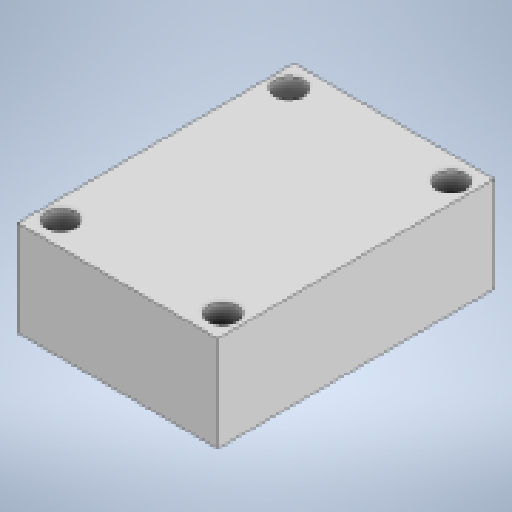
# Autodesk Inventor part: Servo_Driver
Saved by Autodesk Inventor 2025.2 (Build 292293000, 293)
## iProperties
Created: 2025-05-14
Part Number: Servo_Driver
Material: Generic
Document SubType Name: Modeling
Designer: chris
Density: 1 g/cm^3
Appearance: Default
Author: chris
Autodesk Inventor part; units mm, degrees
ref_plane "YZ Plane" through (0, 0, 0) normal (1, 0, 0) x (0, 1, 0)
ref_plane "XZ Plane" through (0, 0, 0) normal (0, 1, 0) x (-1, 0, 0)
ref_plane "XY Plane" through (0, 0, 0) normal (0, 0, 1) x (1, 0, 0)
sketch "Sketch1" plane through (0, 0, 0) normal (0, 1, 0) x (-1, 0, 0)
  line L0 (0, 0) -> (42, 0)
  line L1 (42, 0) -> (42, -58)
  line L2 (42, -58) -> (0, -58)
  line L3 (0, -58) -> (0, 0)
  dimension "d0" = 58
  dimension "d1" = 42
  constraints: 8 end point, 2 parallel, 1 horizontal, 1 perpendicular
  measures "d0" distance of L0.end L1.end
  measures "d1" distance of L1.end L2.end
extrude "Extrusion1" add sketch "Sketch1" along normal blind 20
sketch "Sketch2" plane through (0, 20, 0) normal (0, 1, 0) x (1, 0, 0)
  line L0 (-29.2926, 35.5201) -> (-17.3649, 35.5201) construction
  line L1 (-17.3649, 35.5201) -> (-17.3649, 9.1969) construction
  line L2 (-17.3649, 9.1969) -> (-29.2926, 9.1969) construction
  line L3 (-29.2926, 9.1969) -> (-29.2926, 35.5201) construction
  spline S0 degree 2 poles (-27.9624, 31.884) (-28.3424, 31.884) (-28.8757, 32.0428) (-29.1111, 32.1562) knots 0 0 0 1 2 2 2
  line L4 (-29.1111, 32.1562) -> (-29.1111, 32.7405)
  line L5 (-29.1111, 32.7405) -> (-29.077, 32.7405)
  spline S1 degree 2 poles (-29.077, 32.7405) (-28.8473, 32.525) (-28.2658, 32.2867) (-27.9964, 32.2867) knots 0 0 0 1 2 2 2
  spline S2 degree 2 poles (-27.9964, 32.2867) (-27.6107, 32.2867) (-27.2164, 32.6072) (-27.2164, 32.871) knots 0 0 0 1 2 2 2
  spline S3 degree 2 poles (-27.2164, 32.871) (-27.2164, 33.0809) (-27.4235, 33.3418) (-27.6475, 33.4071) knots 0 0 0 1 2 2 2
  spline S4 degree 2 poles (-27.6475, 33.4071) (-27.8092, 33.4524) (-28.0787, 33.5148) (-28.28, 33.5659) knots 0 0 0 1 2 2 2
  spline S5 degree 2 poles (-28.28, 33.5659) (-28.4616, 33.6141) (-28.748, 33.7588) (-28.8586, 33.875) knots 0 0 0 1 2 2 2
  spline S6 degree 2 poles (-28.8586, 33.875) (-28.9664, 33.9913) (-29.0855, 34.3033) (-29.0855, 34.5075) knots 0 0 0 1 2 2 2
  spline S7 degree 2 poles (-29.0855, 34.5075) (-29.0855, 34.933) (-28.4218, 35.5088) (-27.9085, 35.5088) knots 0 0 0 1 2 2 2
  spline S8 degree 2 poles (-27.9085, 35.5088) (-27.6135, 35.5088) (-27.0916, 35.3925) (-26.8675, 35.2819) knots 0 0 0 1 2 2 2
  line L6 (-26.8675, 35.2819) -> (-26.8675, 34.7259)
  line L7 (-26.8675, 34.7259) -> (-26.9016, 34.7259)
  spline S9 degree 2 poles (-26.9016, 34.7259) (-27.0689, 34.8791) (-27.5908, 35.106) (-27.8773, 35.106) knots 0 0 0 1 2 2 2
  spline S10 degree 2 poles (-27.8773, 35.106) (-28.2006, 35.106) (-28.6005, 34.8025) (-28.6005, 34.5558) knots 0 0 0 1 2 2 2
  spline S11 degree 2 poles (-28.6005, 34.5558) (-28.6005, 34.3345) (-28.3651, 34.0707) (-28.1439, 34.0112) knots 0 0 0 1 2 2 2
  spline S12 degree 2 poles (-28.1439, 34.0112) (-27.9964, 33.9715) (-27.5681, 33.8694) (-27.4263, 33.8268) knots 0 0 0 1 2 2 2
  spline S13 degree 2 poles (-27.4263, 33.8268) (-27.0661, 33.7162) (-26.7314, 33.2709) (-26.7314, 32.9447) knots 0 0 0 1 2 2 2
  spline S14 degree 2 poles (-26.7314, 32.9447) (-26.7314, 32.7377) (-26.8987, 32.3406) (-27.0491, 32.2016) knots 0 0 0 1 2 2 2
  spline S15 degree 2 poles (-27.0491, 32.2016) (-27.2164, 32.0485) (-27.6419, 31.884) (-27.9624, 31.884) knots 0 0 0 1 2 2 2
  line L8 (-26.2577, 31.9464) -> (-26.2577, 35.4464)
  line L9 (-26.2577, 35.4464) -> (-24.0681, 35.4464)
  line L10 (-24.0681, 35.4464) -> (-24.0681, 35.0323)
  line L11 (-24.0681, 35.0323) -> (-25.7926, 35.0323)
  line L12 (-25.7926, 35.0323) -> (-25.7926, 34.0736)
  line L13 (-25.7926, 34.0736) -> (-24.1844, 34.0736)
  line L14 (-24.1844, 34.0736) -> (-24.1844, 33.6595)
  line L15 (-24.1844, 33.6595) -> (-25.7926, 33.6595)
  line L16 (-25.7926, 33.6595) -> (-25.7926, 32.3605)
  line L17 (-25.7926, 32.3605) -> (-24.0681, 32.3605)
  line L18 (-24.0681, 32.3605) -> (-24.0681, 31.9464)
  line L19 (-24.0681, 31.9464) -> (-26.2577, 31.9464)
  line L20 (-20.8489, 31.9464) -> (-21.453, 31.9464)
  line L21 (-21.453, 31.9464) -> (-22.5592, 33.339)
  line L22 (-22.5592, 33.339) -> (-23.0924, 33.339)
  line L23 (-23.0924, 33.339) -> (-23.0924, 31.9464)
  line L24 (-23.0924, 31.9464) -> (-23.5576, 31.9464)
  line L25 (-23.5576, 31.9464) -> (-23.5576, 35.4464)
  line L26 (-23.5576, 35.4464) -> (-22.6556, 35.4464)
  spline S16 degree 2 poles (-22.6556, 35.4464) (-22.355, 35.4464) (-21.9494, 35.3811) (-21.765, 35.262) knots 0 0 0 1 2 2 2
  spline S17 degree 2 poles (-21.765, 35.262) (-21.5807, 35.1429) (-21.368, 34.7713) (-21.368, 34.4962) knots 0 0 0 1 2 2 2
  spline S18 degree 2 poles (-21.368, 34.4962) (-21.368, 34.1133) (-21.7594, 33.5943) (-22.094, 33.4695) knots 0 0 0 1 2 2 2
  line L27 (-22.094, 33.4695) -> (-20.8489, 31.9464)
  spline S19 degree 2 poles (-21.853, 34.4593) (-21.853, 34.6125) (-21.9607, 34.8479) (-22.0742, 34.9245) knots 0 0 0 1 2 2 2
  spline S20 degree 2 poles (-22.0742, 34.9245) (-22.1735, 34.9897) (-22.4372, 35.0436) (-22.6301, 35.0436) knots 0 0 0 1 2 2 2
  line L28 (-22.6301, 35.0436) -> (-23.0924, 35.0436)
  line L29 (-23.0924, 35.0436) -> (-23.0924, 33.7276)
  line L30 (-23.0924, 33.7276) -> (-22.684, 33.7276)
  spline S21 degree 2 poles (-22.684, 33.7276) (-22.4826, 33.7276) (-22.1621, 33.7985) (-22.0515, 33.9091) knots 0 0 0 1 2 2 2
  spline S22 degree 2 poles (-22.0515, 33.9091) (-21.9494, 34.0055) (-21.853, 34.2778) (-21.853, 34.4593) knots 0 0 0 1 2 2 2
  line L31 (-18.0325, 35.4464) -> (-19.2379, 31.9464)
  line L32 (-19.2379, 31.9464) -> (-19.7399, 31.9464)
  line L33 (-19.7399, 31.9464) -> (-20.9453, 35.4464)
  line L34 (-20.9453, 35.4464) -> (-20.4462, 35.4464)
  line L35 (-20.4462, 35.4464) -> (-19.4761, 32.5391)
  line L36 (-19.4761, 32.5391) -> (-18.5061, 35.4464)
  line L37 (-18.5061, 35.4464) -> (-18.0325, 35.4464)
  spline S23 degree 2 poles (-15.2217, 35.0464) (-15.0231, 34.8139) (-14.8019, 34.1331) (-14.8019, 33.6964) knots 0 0 0 1 2 2 2
  spline S24 degree 2 poles (-14.8019, 33.6964) (-14.8019, 33.2709) (-15.0175, 32.5817) (-15.2217, 32.3491) knots 0 0 0 1 2 2 2
  spline S25 degree 2 poles (-15.2217, 32.3491) (-15.4372, 32.1052) (-16.0073, 31.8726) (-16.3505, 31.8726) knots 0 0 0 1 2 2 2
  spline S26 degree 2 poles (-16.3505, 31.8726) (-16.7051, 31.8726) (-17.2723, 32.1137) (-17.4794, 32.3491) knots 0 0 0 1 2 2 2
  spline S27 degree 2 poles (-17.4794, 32.3491) (-17.6808, 32.5817) (-17.8963, 33.2652) (-17.8963, 33.6964) knots 0 0 0 1 2 2 2
  spline S28 degree 2 poles (-17.8963, 33.6964) (-17.8963, 34.136) (-17.6779, 34.8054) (-17.4765, 35.0464) knots 0 0 0 1 2 2 2
  spline S29 degree 2 poles (-17.4765, 35.0464) (-17.2723, 35.279) (-16.7022, 35.5201) (-16.3505, 35.5201) knots 0 0 0 1 2 2 2
  spline S30 degree 2 poles (-16.3505, 35.5201) (-15.9932, 35.5201) (-15.4202, 35.2705) (-15.2217, 35.0464) knots 0 0 0 1 2 2 2
  spline S31 degree 2 poles (-15.2869, 33.6964) (-15.2869, 34.0424) (-15.4372, 34.5784) (-15.5734, 34.7543) knots 0 0 0 1 2 2 2
  spline S32 degree 2 poles (-15.5734, 34.7543) (-15.7124, 34.9358) (-16.1038, 35.1173) (-16.3477, 35.1173) knots 0 0 0 1 2 2 2
  spline S33 degree 2 poles (-16.3477, 35.1173) (-16.6001, 35.1173) (-16.9802, 34.9415) (-17.1248, 34.7543) knots 0 0 0 1 2 2 2
  spline S34 degree 2 poles (-17.1248, 34.7543) (-17.2638, 34.5756) (-17.4113, 34.0367) (-17.4113, 33.6964) knots 0 0 0 1 2 2 2
  spline S35 degree 2 poles (-17.4113, 33.6964) (-17.4113, 33.0071) (-16.8327, 32.2754) (-16.3477, 32.2754) knots 0 0 0 1 2 2 2
  spline S36 degree 2 poles (-16.3477, 32.2754) (-15.8627, 32.2754) (-15.2869, 33.0071) (-15.2869, 33.6964) knots 0 0 0 1 2 2 2
  spline S37 degree 2 poles (-26.1783, 27.9309) (-26.1783, 27.4515) (-26.5669, 26.6801) (-26.8931, 26.4645) knots 0 0 0 1 2 2 2
  spline S38 degree 2 poles (-26.8931, 26.4645) (-27.1597, 26.2972) (-27.7071, 26.1837) (-28.1325, 26.1837) knots 0 0 0 1 2 2 2
  line L38 (-28.1325, 26.1837) -> (-28.9381, 26.1837)
  line L39 (-28.9381, 26.1837) -> (-28.9381, 29.6837)
  line L40 (-28.9381, 29.6837) -> (-28.141, 29.6837)
  spline S39 degree 2 poles (-28.141, 29.6837) (-27.6475, 29.6837) (-27.0859, 29.5362) (-26.8874, 29.4057) knots 0 0 0 1 2 2 2
  spline S40 degree 2 poles (-26.8874, 29.4057) (-26.5499, 29.1817) (-26.1783, 28.4414) (-26.1783, 27.9309) knots 0 0 0 1 2 2 2
  spline S41 degree 2 poles (-26.6633, 27.9365) (-26.6633, 28.3393) (-26.9299, 28.9094) (-27.1937, 29.0711) knots 0 0 0 1 2 2 2
  spline S42 degree 2 poles (-27.1937, 29.0711) (-27.3809, 29.1817) (-27.8035, 29.2809) (-28.1184, 29.2809) knots 0 0 0 1 2 2 2
  line L41 (-28.1184, 29.2809) -> (-28.4729, 29.2809)
  line L42 (-28.4729, 29.2809) -> (-28.4729, 26.5865)
  line L43 (-28.4729, 26.5865) -> (-28.1184, 26.5865)
  spline S43 degree 2 poles (-28.1184, 26.5865) (-27.8092, 26.5865) (-27.3412, 26.6857) (-27.1512, 26.819) knots 0 0 0 1 2 2 2
  spline S44 degree 2 poles (-27.1512, 26.819) (-26.9073, 26.9835) (-26.6633, 27.5281) (-26.6633, 27.9365) knots 0 0 0 1 2 2 2
  line L44 (-22.9648, 26.1837) -> (-23.5689, 26.1837)
  line L45 (-23.5689, 26.1837) -> (-24.6751, 27.5763)
  line L46 (-24.6751, 27.5763) -> (-25.2083, 27.5763)
  line L47 (-25.2083, 27.5763) -> (-25.2083, 26.1837)
  line L48 (-25.2083, 26.1837) -> (-25.6735, 26.1837)
  line L49 (-25.6735, 26.1837) -> (-25.6735, 29.6837)
  line L50 (-25.6735, 29.6837) -> (-24.7715, 29.6837)
  spline S45 degree 2 poles (-24.7715, 29.6837) (-24.4709, 29.6837) (-24.0653, 29.6185) (-23.8809, 29.4993) knots 0 0 0 1 2 2 2
  spline S46 degree 2 poles (-23.8809, 29.4993) (-23.6966, 29.3802) (-23.4838, 29.0087) (-23.4838, 28.7335) knots 0 0 0 1 2 2 2
  spline S47 degree 2 poles (-23.4838, 28.7335) (-23.4838, 28.3506) (-23.8752, 27.8316) (-24.2099, 27.7068) knots 0 0 0 1 2 2 2
  line L51 (-24.2099, 27.7068) -> (-22.9648, 26.1837)
  spline S48 degree 2 poles (-23.9688, 28.6967) (-23.9688, 28.8498) (-24.0766, 29.0852) (-24.1901, 29.1618) knots 0 0 0 1 2 2 2
  spline S49 degree 2 poles (-24.1901, 29.1618) (-24.2893, 29.2271) (-24.5531, 29.2809) (-24.746, 29.2809) knots 0 0 0 1 2 2 2
  line L52 (-24.746, 29.2809) -> (-25.2083, 29.2809)
  line L53 (-25.2083, 29.2809) -> (-25.2083, 27.9649)
  line L54 (-25.2083, 27.9649) -> (-24.7999, 27.9649)
  spline S50 degree 2 poles (-24.7999, 27.9649) (-24.5985, 27.9649) (-24.278, 28.0358) (-24.1674, 28.1464) knots 0 0 0 1 2 2 2
  spline S51 degree 2 poles (-24.1674, 28.1464) (-24.0653, 28.2429) (-23.9688, 28.5151) (-23.9688, 28.6967) knots 0 0 0 1 2 2 2
  line L55 (-21.4672, 26.1837) -> (-22.823, 26.1837)
  line L56 (-22.823, 26.1837) -> (-22.823, 26.5411)
  line L57 (-22.823, 26.5411) -> (-22.3777, 26.5411)
  line L58 (-22.3777, 26.5411) -> (-22.3777, 29.3263)
  line L59 (-22.3777, 29.3263) -> (-22.823, 29.3263)
  line L60 (-22.823, 29.3263) -> (-22.823, 29.6837)
  line L61 (-22.823, 29.6837) -> (-21.4672, 29.6837)
  line L62 (-21.4672, 29.6837) -> (-21.4672, 29.3263)
  line L63 (-21.4672, 29.3263) -> (-21.9125, 29.3263)
  line L64 (-21.9125, 29.3263) -> (-21.9125, 26.5411)
  line L65 (-21.9125, 26.5411) -> (-21.4672, 26.5411)
  line L66 (-21.4672, 26.5411) -> (-21.4672, 26.1837)
  line L67 (-18.353, 29.6837) -> (-19.5584, 26.1837)
  line L68 (-19.5584, 26.1837) -> (-20.0604, 26.1837)
  line L69 (-20.0604, 26.1837) -> (-21.2658, 29.6837)
  line L70 (-21.2658, 29.6837) -> (-20.7667, 29.6837)
  line L71 (-20.7667, 29.6837) -> (-19.7966, 26.7765)
  line L72 (-19.7966, 26.7765) -> (-18.8266, 29.6837)
  line L73 (-18.8266, 29.6837) -> (-18.353, 29.6837)
  line L74 (-18.0183, 26.1837) -> (-18.0183, 29.6837)
  line L75 (-18.0183, 29.6837) -> (-15.8287, 29.6837)
  line L76 (-15.8287, 29.6837) -> (-15.8287, 29.2696)
  line L77 (-15.8287, 29.2696) -> (-17.5531, 29.2696)
  line L78 (-17.5531, 29.2696) -> (-17.5531, 28.3109)
  line L79 (-17.5531, 28.3109) -> (-15.9449, 28.3109)
  line L80 (-15.9449, 28.3109) -> (-15.9449, 27.8968)
  line L81 (-15.9449, 27.8968) -> (-17.5531, 27.8968)
  line L82 (-17.5531, 27.8968) -> (-17.5531, 26.5978)
  line L83 (-17.5531, 26.5978) -> (-15.8287, 26.5978)
  line L84 (-15.8287, 26.5978) -> (-15.8287, 26.1837)
  line L85 (-15.8287, 26.1837) -> (-18.0183, 26.1837)
  line L86 (-12.6094, 26.1837) -> (-13.2136, 26.1837)
  line L87 (-13.2136, 26.1837) -> (-14.3197, 27.5763)
  line L88 (-14.3197, 27.5763) -> (-14.853, 27.5763)
  line L89 (-14.853, 27.5763) -> (-14.853, 26.1837)
  line L90 (-14.853, 26.1837) -> (-15.3181, 26.1837)
  line L91 (-15.3181, 26.1837) -> (-15.3181, 29.6837)
  line L92 (-15.3181, 29.6837) -> (-14.4162, 29.6837)
  spline S52 degree 2 poles (-14.4162, 29.6837) (-14.1155, 29.6837) (-13.7099, 29.6185) (-13.5256, 29.4993) knots 0 0 0 1 2 2 2
  spline S53 degree 2 poles (-13.5256, 29.4993) (-13.3412, 29.3802) (-13.1285, 29.0087) (-13.1285, 28.7335) knots 0 0 0 1 2 2 2
  spline S54 degree 2 poles (-13.1285, 28.7335) (-13.1285, 28.3506) (-13.5199, 27.8316) (-13.8546, 27.7068) knots 0 0 0 1 2 2 2
  line L93 (-13.8546, 27.7068) -> (-12.6094, 26.1837)
  spline S55 degree 2 poles (-13.6135, 28.6967) (-13.6135, 28.8498) (-13.7213, 29.0852) (-13.8347, 29.1618) knots 0 0 0 1 2 2 2
  spline S56 degree 2 poles (-13.8347, 29.1618) (-13.934, 29.2271) (-14.1978, 29.2809) (-14.3906, 29.2809) knots 0 0 0 1 2 2 2
  line L94 (-14.3906, 29.2809) -> (-14.853, 29.2809)
  line L95 (-14.853, 29.2809) -> (-14.853, 27.9649)
  line L96 (-14.853, 27.9649) -> (-14.4445, 27.9649)
  spline S57 degree 2 poles (-14.4445, 27.9649) (-14.2432, 27.9649) (-13.9227, 28.0358) (-13.812, 28.1464) knots 0 0 0 1 2 2 2
  spline S58 degree 2 poles (-13.812, 28.1464) (-13.7099, 28.2429) (-13.6135, 28.5151) (-13.6135, 28.6967) knots 0 0 0 1 2 2 2
  point P0 (0, 0)
  constraints: 2 other
extrude "Extrusion2" add sketch "Sketch2" against normal blind 1
sketch "Sketch5" plane through (0, 20, 0) normal (0, 1, 0) x (1, 0, 0)
  circle A0 centre (-4, 53) radius 1.55
  circle A1 centre (-38, 53) radius 1.55
  circle A2 centre (-38, 5) radius 1.55
  circle A3 centre (-4, 5) radius 1.55
  line L0 (-42, 58) -> (-42, 0) projected
  line L1 (-42, 0) -> (0, 0) projected
  dimension "d6" = 3.1
  dimension "d7" = 3.1
  dimension "d8" = 3.1
  dimension "d9" = 3.1
  dimension "d10" = 34
  dimension "d11" = 48
  dimension "d12" = 48
  dimension "d13" = 34
  dimension "d14" = 0
  dimension "d15" = 0
  dimension "d16" = 4
  dimension "d17" = 5
  constraints: 4 centre point
  measures "d6" diameter of A0
  measures "d7" diameter of A1
  measures "d8" diameter of A2
  measures "d9" diameter of A3
  measures "d10" distance of A3.centre A2.centre
  measures "d11" distance of A1.centre A2.centre
  measures "d12" distance of A0.centre A3.centre
  measures "d13" distance of A0.centre A1.centre
  measures "d14" vertical distance of A3.centre A2.centre
  measures "d15" horizontal distance of A1.centre A2.centre
  measures "d16" distance from line of L0 A2.centre
  measures "d17" distance from line of L1 A2.centre
hole "Hole1" at (-38, 20, -53) at (-38, 20, -5) at (-4, 20, -5) at (-4, 20, -53) direction (0, -1, 0) diameter 3.1 end through all
sketch "Sketch6" plane through (0, 20, 0) normal (0, 1, 0) x (1, 0, 0)
  circle A0 centre (-4, 5) radius 3
  circle A1 centre (-4, 53) radius 3
  circle A2 centre (-38, 53) radius 3
  circle A3 centre (-38, 5) radius 3
  circle A4 centre (-4, 5) radius 1.55 projected
  circle A5 centre (-38, 5) radius 1.55 projected
  circle A6 centre (-38, 53) radius 1.55 projected
  circle A7 centre (-4, 53) radius 1.55 projected
  circle A8 centre (-4, 53) radius 1.55
  circle A9 centre (-38, 5) radius 1.55
  circle A10 centre (-4, 5) radius 1.55
  circle A11 centre (-38, 53) radius 1.55
  point P0 (0, 0)
  dimension "d25" = 6
  dimension "d26" = 6
  dimension "d27" = 6
  dimension "d28" = 6
  dimension "d29" = 3.1
  dimension "d30" = 3.1
  dimension "d31" = 3.1
  dimension "d32" = 3.1
  constraints: 8 centre point, 8 concentric
  measures "d25" diameter of A0
  measures "d26" diameter of A1
  measures "d27" diameter of A2
  measures "d28" diameter of A3
  measures "d29" diameter of A8
  measures "d30" diameter of A9
  measures "d31" diameter of A10
  measures "d32" diameter of A11
extrude "Extrusion3" cut sketch "Sketch6" against normal blind 18.5
equation "\"d12\" = d11"
equation "\"d13\" = d10"
body "Solid1"
